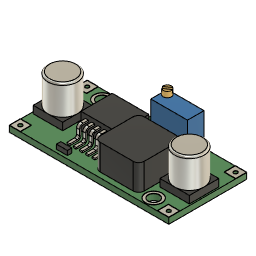
LM2596 v1 (Autodesk Fusion 360 design; units mm, degrees)
Autodesk Fusion 360 part; units mm, degrees
note: some values were not read from the file. Set by a fixed rule: which sketch regions a step uses.
sketch "Sketch1" plane through (0, 0, 0) normal (0, 0, 1) x (1, 0, 0) in component "LM2596_Module"
  line L0 (0, 0) -> (43.4, 0)
  line L1 (43.4, 0) -> (43.4, 21.2)
  line L2 (43.4, 21.2) -> (0, 21.2)
  line L3 (0, 21.2) -> (0, 0)
  circle A0 centre (1.5, 1.5) radius 0.5
  circle A1 centre (1.5, 19.7) radius 0.5
  circle A2 centre (41.9, 19.7) radius 0.5
  circle A3 centre (41.9, 1.5) radius 0.5
  circle A4 centre (36.8, 2.5) radius 1.5
  circle A5 centre (6.6, 18.7) radius 1.5
  circle A6 centre (6.6, 18.7) radius 2.25
  circle A7 centre (36.8, 2.5) radius 2.25
  circle A8 centre (4.5, 10) radius 4
  circle A9 centre (39, 10) radius 4
  line L4 (0.5, 14) -> (8.5, 14)
  line L5 (8.5, 14) -> (8.5, 6)
  line L6 (8.5, 6) -> (0.5, 6)
  line L7 (0.5, 6) -> (0.5, 14)
  line L8 (35, 14) -> (43, 14)
  line L9 (43, 14) -> (43, 6)
  line L10 (43, 6) -> (35, 6)
  line L11 (35, 6) -> (35, 14)
  line L12 (23.3, 13.4) -> (32.3, 13.4)
  line L13 (33.8, 11.9) -> (33.8, 2.9)
  line L14 (32.3, 1.4) -> (23.3, 1.4)
  line L15 (21.8, 2.9) -> (21.8, 11.9)
  arc A10 (23.3, 13.4) -> (21.8, 11.9) centre (23.3, 11.9) ccw
  arc A11 (33.8, 11.9) -> (32.3, 13.4) centre (32.3, 11.9) ccw
  arc A12 (32.3, 1.4) -> (33.8, 2.9) centre (32.3, 2.9) ccw
  arc A13 (21.8, 2.9) -> (23.3, 1.4) centre (23.3, 2.9) ccw
  line L16 (23, 20) -> (33, 20)
  line L17 (33, 20) -> (33, 15.5)
  line L18 (33, 15.5) -> (23, 15.5)
  line L19 (23, 15.5) -> (23, 20)
  line L20 (23, 15.5) -> (24, 15.5)
  line L21 (24, 15.5) -> (24, 15)
  line L22 (24, 15) -> (23, 15)
  line L23 (23, 15) -> (23, 15.5)
  line L24 (33, 15.5) -> (32, 15.5)
  line L25 (32, 15.5) -> (32, 15)
  line L26 (32, 15) -> (33, 15)
  line L27 (33, 15) -> (33, 15.5)
  line L28 (3, 18) -> (0, 18)
  line L29 (0, 18) -> (0, 21.2)
  line L30 (0, 21.2) -> (3, 21.2)
  line L31 (3, 21.2) -> (3, 18)
  line L32 (3, 3) -> (0, 3)
  line L33 (0, 3) -> (0, 0)
  line L34 (0, 0) -> (3, 0)
  line L35 (3, 0) -> (3, 3)
  line L36 (40.3, 3) -> (43.4, 3)
  line L37 (43.4, 3) -> (43.4, 0)
  line L38 (43.4, 0) -> (40.3, 0)
  line L39 (40.3, 0) -> (40.3, 3)
  line L40 (40.3, 18.2) -> (43.4, 18.2)
  line L41 (43.4, 18.2) -> (43.4, 21.2)
  line L42 (43.4, 21.2) -> (40.3, 21.2)
  line L43 (40.3, 21.2) -> (40.3, 18.2)
  line L44 (11, 17) -> (21, 17)
  line L45 (21, 8.5) -> (11, 8.5)
  line L46 (11, 17) -> (21, 17)
  line L47 (21, 18.7) -> (11, 18.7)
  line L48 (21, 8.5) -> (21, 18.7)
  line L49 (11, 8.5) -> (11, 18.7)
  line L50 (19, 8.5) -> (19.8, 8.5)
  line L51 (19.8, 8.5) -> (19.8, 3.5)
  line L52 (19.8, 3.5) -> (19, 3.5)
  line L53 (19, 3.5) -> (19, 8.5)
  line L54 (12.2, 3.5) -> (12.2, 8.5)
  line L55 (12.2, 8.5) -> (13, 8.5)
  line L56 (13, 8.5) -> (13, 3.5)
  line L57 (13, 3.5) -> (12.2, 3.5)
  line L58 (15.6, 3.5) -> (15.6, 8.5)
  line L59 (15.6, 8.5) -> (16.4, 8.5)
  line L60 (16.4, 8.5) -> (16.4, 3.5)
  line L61 (16.4, 3.5) -> (15.6, 3.5)
  line L62 (13.9, 3.5) -> (13.9, 8.5)
  line L63 (13.9, 8.5) -> (14.7, 8.5)
  line L64 (14.7, 8.5) -> (14.7, 3.5)
  line L65 (14.7, 3.5) -> (13.9, 3.5)
  line L66 (17.3, 3.5) -> (17.3, 8.5)
  line L67 (17.3, 8.5) -> (18.1, 8.5)
  line L68 (18.1, 8.5) -> (18.1, 3.5)
  line L69 (18.1, 3.5) -> (17.3, 3.5)
  line L70 (12, 2) -> (15, 2)
  line L71 (15, 2) -> (15, 0.8)
  line L72 (15, 0.8) -> (12, 0.8)
  line L73 (12, 0.8) -> (12, 2)
  line L74 (12.2, 6.5) -> (13, 6.5)
  line L75 (13, 6.1) -> (12.2, 6.1)
  line L76 (14.7, 6.1) -> (13.9, 6.1)
  line L77 (13.9, 6.5) -> (14.7, 6.5)
  line L78 (15.6, 6.5) -> (16.4, 6.5)
  line L79 (16.4, 6.1) -> (15.6, 6.1)
  line L80 (19.8, 6.1) -> (19, 6.1)
  line L81 (18.1, 6.1) -> (17.3, 6.1)
  line L82 (17.3, 6.5) -> (18.1, 6.5)
  line L83 (19, 6.5) -> (19.8, 6.5)
  circle A14 centre (24.2, 18.8) radius 1.1
  line L84 (23.5052, 17.9472) -> (25.239, 19.1613)
  line L85 (24.8099, 19.7154) -> (23.1312, 18.5399)
  line L86 (6.6, 18.7) -> (36.8, 18.7) construction
  line L87 (36.8, 18.7) -> (36.8, 2.5) construction
  line L88 (36.8, 2.5) -> (6.6, 2.5) construction
  line L89 (6.6, 2.5) -> (6.6, 18.7) construction
  dimension "d1" = 43.4
  dimension "d2" = 21.2
  dimension "d24" = 8
  dimension "d25" = 8
  dimension "d32" = 10
  dimension "d39" = 3
  dimension "d40" = 1.2
  dimension "d69" = 2.2
  dimension "d82" = 30.2
  dimension "d83" = 16.2
  constraint horizontal L0
  constraint vertical L1
  constraint horizontal L2
  constraint vertical L3
  constraint coincident L0.start L3.end
  constraint concentric A5 A6
  constraint concentric A4 A7
  constraint horizontal L4
  constraint vertical L5
  constraint horizontal L6
  constraint vertical L7
  constraint horizontal L8
  constraint vertical L9
  constraint horizontal L10
  constraint vertical L11
  constraint vertical L13
  constraint horizontal L16
  constraint vertical L17
  constraint horizontal L18
  constraint vertical L19
  constraint horizontal L20
  constraint vertical L21
  constraint horizontal L22
  constraint vertical L23
  constraint horizontal L24
  constraint vertical L25
  constraint horizontal L26
  constraint vertical L27
  constraint horizontal L28
  constraint vertical L29
  constraint horizontal L30
  constraint vertical L31
  constraint horizontal L32
  constraint vertical L33
  constraint horizontal L34
  constraint vertical L35
  constraint horizontal L36
  constraint vertical L37
  constraint horizontal L38
  constraint vertical L39
  constraint horizontal L40
  constraint vertical L41
  constraint horizontal L42
  constraint vertical L43
  constraint horizontal L44
  constraint horizontal L45
  constraint horizontal L46
  constraint horizontal L47
  constraint perpendicular L47 L49
  constraint coincident L44.end L48
  constraint horizontal L50
  constraint vertical L51
  constraint horizontal L52
  constraint vertical L53
  constraint horizontal L55
  constraint vertical L56
  constraint horizontal L57
  constraint vertical L54
  constraint horizontal L59
  constraint vertical L60
  constraint horizontal L61
  constraint vertical L58
  constraint horizontal L63
  constraint vertical L64
  constraint horizontal L65
  constraint vertical L62
  constraint horizontal L67
  constraint vertical L68
  constraint horizontal L69
  constraint vertical L66
  constraint horizontal L70
  constraint vertical L71
  constraint horizontal L72
  constraint vertical L73
  constraint coincident L51 L83.end
  constraint perpendicular L51 L74
  constraint coincident L54 L75.end
  constraint perpendicular L54 L80
  constraint coincident L54 L74.start
  constraint coincident L56 L74.end
  constraint coincident L62 L77.start
  constraint collinear L74 L77
  constraint coincident L62 L76.end
  constraint coincident L56 L75.start
  constraint collinear L75 L80
  constraint coincident L58 L79.end
  constraint coincident L64 L76.start
  constraint collinear L76 L80
  constraint coincident L64 L77.end
  constraint coincident L58 L78.start
  constraint collinear L77 L78
  constraint coincident L60 L78.end
  constraint coincident L66 L82.start
  constraint collinear L78 L82
  constraint coincident L66 L81.end
  constraint coincident L60 L79.start
  constraint collinear L79 L80
  constraint coincident L53 L80.end
  constraint coincident L68 L81.start
  constraint collinear L80 L81
  constraint coincident L68 L82.end
  constraint coincident L53 L83.start
  constraint collinear L82 L83
  constraint coincident L51 L80.start
  constraint coincident A14 L85.end
  constraint coincident A14 L84.start
  constraint coincident A14 L84.end
  constraint coincident A14 L85.start
  constraint horizontal L86
  constraint vertical L87
  constraint horizontal L88
  constraint vertical L89
  constraint coincident A4.centre A7.centre
  constraint coincident A5.centre A6.centre
  measures "d1" distance of L0.start L0.end
  measures "d2" distance of L0.start L2.end
  measures "d24" diameter of A8
  measures "d25" diameter of A9
  measures "d32" distance of L44.start L44.end
  measures "d39" distance of L70.start L70.end
  measures "d40" distance of L70.start L72.end
  measures "d69" diameter of A14
  measures "d82" distance of A5.centre L86.end
  measures "d83" distance of A5.centre L88.end
extrude "Extrude1" add sketch "Sketch1" against normal blind 1.6 contours L0 L3 L32 L33 L34 L35 | L0 L1 L2 L3 L28 L31 L32 L35 L36 L39 L40 L43 | L0 L1 L36 L37 L38 L39 | L2 L3 L28 L29 L30 L31 | L1 L2 L40 L41 L42 L43 | A6 | A7 | A8 | A8 L5 L6 | A8 L4 L5 | A8 L4 L7 | A8 L6 L7 | A9 | A9 L9 L10 | A9 L8 L9 | A9 L8 L11 | A9 L10 L11 | L12 L13 L14 L15 A10 A11 A12 A13 | L16 L17 L18 L19 L20 L24 | L18 L20 L21 L22 L23 | L18 L24 L25 L26 L27 | L44 L46 L47 L48 L49 | L44 L45 L46 L48 L49 L50 L55 L59 L63 L67 | L45 L54 L55 L56 L74 | L45 L50 L51 L53 L83 | L54 L56 L74 L75 | L51 L53 L80 L83 | L45 L62 L63 L64 L77 | L54 L56 L57 L75 | L45 L66 L67 L68 L82 | L51 L52 L53 L80 | L62 L64 L76 L77 | L66 L68 L81 L82 | L45 L58 L59 L60 L78 | L62 L64 L65 L76 | L66 L68 L69 L81 | L58 L60 L78 L79 | L58 L60 L61 L79 | L70 L71 L72 L73 | A14 L84 | A14 L84 L85 | A14 L85 makes body 1 in component "LM2596_Module"
extrude "Extrude2" add sketch "Sketch1" along normal blind 0.1 separate body contours L0 L3 L32 L33 L34 L35 | L0 L1 L36 L37 L38 L39 | L2 L3 L28 L29 L30 L31 | L1 L2 L40 L41 L42 L43 | A6 | A7 makes body 2 at (35.4161, 3.9366, 0) makes body 3 at (1.5125, 18.4005, 0) makes body 4 at (40.6667, 19.7, 0) makes body 5 at (40.6667, 1.5, 0) makes body 6 at (1.5125, 2.6662, 0) makes body 7 at (8.586, 18.5137, 0) in component "LM2596_Module"
extrude "Extrude3" add sketch "Sketch1" along normal blind 2 separate body contours A8 | A8 L5 L6 | A8 L4 L5 | A8 L4 L7 | A8 L6 L7 | A9 | A9 L9 L10 | A9 L8 L9 | A9 L8 L11 | A9 L10 L11 makes body 8 at (5.8333, 8.6667, 0) makes body 9 at (37.6667, 11.3333, 0) in component "LM2596_Module"
extrude "Extrude4" add sketch "Sketch1" along normal blind 10 contours A8 | A9 bodies 8 9 in component "LM2596_Module"
extrude "Extrude5" add sketch "Sketch1" along normal blind 4.6 separate body contours L44 L45 L46 L48 L49 L50 L55 L59 L63 L67 makes body 10 in component "LM2596_Module"
extrude "Extrude6" add sketch "Sketch1" along normal blind 1 separate body contours L44 L46 L47 L48 L49 makes body 11 in component "LM2596_Module"
extrude "Extrude7" add sketch "Sketch1" along normal blind 0.4 separate body contours L54 L56 L57 L75 | L51 L52 L53 L80 | L62 L64 L65 L76 | L66 L68 L69 L81 | L58 L60 L61 L79 makes body 12 at (15.8667, 5.2333, 0) makes body 13 at (14.1667, 5.2333, 0) makes body 14 at (17.5667, 5.2333, 0) makes body 15 at (12.4667, 5.2333, 0) makes body 16 at (19.2667, 5.2333, 0) in component "LM2596_Module"
extrude "Extrude8" add sketch "Sketch1" along normal blind 3.5 contours L54 L56 L74 L75 | L51 L53 L80 L83 | L62 L64 L76 L77 | L66 L68 L81 L82 | L58 L60 L78 L79 bodies 12 13 14 15 16 in component "LM2596_Module"
extrude "Extrude9" add sketch "Sketch1" along normal blind 3.5 and the other way blind -3.1 contours L45 L54 L55 L56 L74 | L45 L50 L51 L53 L83 | L45 L62 L63 L64 L77 | L45 L66 L67 L68 L82 | L45 L58 L59 L60 L78 bodies 12 13 14 15 16 in component "LM2596_Module"
fillet "Fillet1" radius 1 10 edges at (16, 6.1, 3.5) (16, 6.5, 0) (14.3, 6.1, 3.5) (14.3, 6.5, 0) (17.7, 6.1, 3.5) (17.7, 6.5, 0) (12.6, 6.1, 3.5) (12.6, 6.5, 0) (19.4, 6.1, 3.5) (19.4, 6.5, 0) on bodies 12 13 14 15 16 in component "LM2596_Module"
fillet "Fillet2" radius 0.6 10 edges at (16, 6.5, 3.1) (16, 6.1, 0.4) (14.3, 6.5, 3.1) (14.3, 6.1, 0.4) (17.7, 6.5, 3.1) (17.7, 6.1, 0.4) (12.6, 6.5, 3.1) (12.6, 6.1, 0.4) (19.4, 6.5, 3.1) (19.4, 6.1, 0.4) on bodies 12 13 14 15 16 in component "LM2596_Module"
extrude "Extrude10" add sketch "Sketch1" along normal blind 7 separate body contours L12 L13 L14 L15 A10 A11 A12 A13 makes body 17 in component "LM2596_Module"
extrude "Extrude11" add sketch "Sketch1" along normal blind 10 separate body contours L16 L17 L18 L19 L20 L24 | A14 L84 | A14 L84 L85 | A14 L85 makes body 18 in component "LM2596_Module"
extrude "Extrude12" add sketch "Sketch1" along normal blind 11.5 and the other way blind -10 separate body contours A14 L84 | A14 L84 L85 | A14 L85 makes body 19 in component "LM2596_Module"
extrude "Extrude13" cut sketch "Sketch1" along normal blind 12.1 and the other way blind -10.7 contours A14 L84 L85 bodies 19 in component "LM2596_Module"
extrude "Extrude14" add sketch "Sketch1" along normal blind 1.2 separate body contours L70 L71 L72 L73 makes body 20 in component "LM2596_Module"
fillet "Fillet3" radius 0.5 2 edges at (0.7707, 8.5535, 10) (35.2707, 8.5535, 10) on bodies 8 9 in component "LM2596_Module"
component "LM2596_Module" placed x (1, 0, 0) y (0, 1, 0) z (0, 0, 1) at (0, 0, 0)
equation "d59 = -3.5 mm + 0.4 mm"
equation "d60 = 0.0 °"
equation "d70 = 10.00 mm + 1.5 mm"
equation "d73 = 0.0 °"
equation "d77 = 0.0 °"
named bodies: "pcb"
